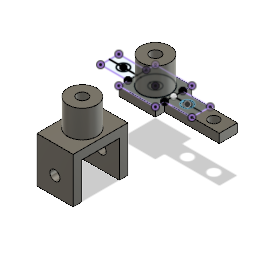
AluminumFesting v3 (Autodesk Fusion 360 design; units mm, degrees)
Autodesk Fusion 360 part; units mm, degrees
sketch "Sketch1" plane through (0, 0, 0) normal (0, 1, 0) x (1, 0, 0)
  line L0 (-10, 10) -> (10, 10)
  line L1 (10, 10) -> (10, -10)
  line L2 (10, -10) -> (-10, -10)
  line L3 (-10, -10) -> (-10, 10)
  line L4 (-10, 10) -> (10, -10) construction
  line L5 (10, 10) -> (-10, -10) construction
  line L6 (-10, -5) -> (-25, -5)
  line L7 (-25, -5) -> (-25, 5)
  line L8 (-25, 5) -> (-10, 5)
  line L9 (-10, 5) -> (-10, -5)
  line L10 (10, -5) -> (25, -5)
  line L11 (25, -5) -> (25, 5)
  line L12 (25, 5) -> (10, 5)
  line L13 (10, 5) -> (10, -5)
  dimension "d1" = 20
  constraint horizontal L0
  constraint perpendicular L0 L1
  constraint parallel L0 L2
  constraint parallel L1 L3
  constraint coincident L4 origin
  constraint coincident L5 origin
  constraint horizontal L6
  constraint vertical L7
  constraint horizontal L8
  constraint vertical L9
  constraint coincident L3 L6.start
  constraint horizontal L10
  constraint vertical L11
  constraint horizontal L12
  constraint vertical L13
  constraint coincident L1 L10.start
  measures "d1" distance of L0.end L1.end
extrude "Extrude1" add sketch "Sketch1" along normal blind 5 makes body 1
sketch "Sketch2" plane through (0, 5, 0) normal (0, 1, 0) x (-1, 0, 0)
  line L0 (-10, 5) -> (-25, 5)
  line L1 (-25, 5) -> (-25, -5)
  line L2 (-25, -5) -> (-10, -5)
  line L3 (-10, -5) -> (-10, -10)
  line L4 (-10, -10) -> (10, -10)
  line L5 (10, -10) -> (10, -5)
  line L6 (10, -5) -> (25, -5)
  line L7 (25, -5) -> (25, 5)
  line L8 (25, 5) -> (10, 5)
  line L9 (10, 5) -> (10, 10)
  line L10 (10, 10) -> (-10, 10)
  line L11 (-10, 10) -> (-10, 5)
  line L12 (10, -5) -> (10, 5)
  line L13 (-10, 5) -> (-10, -5)
  line L14 (10, 0) -> (25, 0)
  line L15 (-10, 0) -> (-25, 0)
  circle A0 centre (17.5, 0) radius 2.75
  circle A1 centre (-17.5, 0) radius 2.75
  circle A2 centre (0, 0) radius 2.9
  circle A3 centre (0, 0) radius 8
  dimension "d4" = 5.5
  dimension "d5" = 5.5
  dimension "d6" = 5.8
  dimension "d7" = 16
  constraint coincident L5.end L6.start
  constraint coincident L8.end L9.start
  constraint coincident L0.start L11.end
  constraint coincident L2.end L3.start
  constraint midpoint L12 L14.start
  constraint midpoint L7 L14.end
  constraint midpoint L1 L15.end
  constraint perpendicular L1 L15
  constraint midpoint L14 A0.centre
  constraint midpoint L15 A1.centre
  constraint coincident A2.centre A3.centre
  measures "d4" diameter of A0
  measures "d5" diameter of A1
  measures "d6" diameter of A2
  measures "d7" diameter of A3
extrude "Extrude2" cut sketch "Sketch2" against normal blind 12 contours L15 A1 | L15 A1 | L14 A0 | L14 A0 bodies 1
extrude "Extrude3" add sketch "Sketch2" along normal blind 15 contours A3 bodies 1
copy_body "CopyPasteBodies1" bodies 1 makes body 2
move_body "Move1" bodies 2 to x (1, 0, 0) y (0, 1, 0) z (0, 0, 1) at (0, 0, 40)
sketch "Sketch3" plane through (0, 5, 0) normal (0, 1, 0) x (-1, 0, 0)
  line L0 (-10, 45) -> (-25, 45)
  line L1 (-25, 45) -> (-25, 35)
  line L2 (-25, 35) -> (-10, 35)
  line L3 (-10, 35) -> (-10, 30)
  line L4 (-10, 30) -> (10, 30)
  line L5 (10, 30) -> (10, 35)
  line L6 (10, 35) -> (25, 35)
  line L7 (25, 35) -> (25, 45)
  line L8 (25, 45) -> (10, 45)
  line L9 (10, 45) -> (10, 50)
  line L10 (10, 50) -> (-10, 50)
  line L11 (-10, 50) -> (-10, 45)
  circle A0 centre (-17.5, 40) radius 2.75
  circle A1 centre (17.5, 40) radius 2.75
  circle A2 centre (0, 40) radius 8
  line L12 (-10, 45) -> (-10, 35)
  line L13 (10, 45) -> (10, 35)
  constraint coincident L0.start L11.end
  constraint coincident L2.end L3.start
  constraint coincident L8.end L9.start
  constraint coincident L5.end L6.start
extrude "Extrude4" cut sketch "Sketch3" against normal blind 25 contours L0 L1 L2 L12 | L6 L7 L8 L13 bodies 2
sketch "Sketch4" plane through (0, 0, 50) normal (0, 0, 1) x (1, 0, 0)
  line L0 (-10, 0) -> (10, 0)
  line L1 (10, 0) -> (10, 5)
  line L2 (10, 5) -> (-10, 5)
  line L3 (-10, 5) -> (-10, 0)
  line L4 (-10, 5) -> (10, 5)
  line L5 (10, 5) -> (10, -20)
  line L6 (10, -20) -> (-10, -20)
  line L7 (-10, -20) -> (-10, 5)
  dimension "d14" = 25
  constraint horizontal L4
  constraint vertical L5
  constraint horizontal L6
  constraint vertical L7
  constraint coincident L2.end L3.start
  measures "d14" distance of L2.end L6.end
extrude "Extrude5" add sketch "Sketch4" along normal blind 5 bodies 2
sketch "Sketch5" plane through (0, 0, 30) normal (0, 0, -1) x (-1, 0, 0)
  line L0 (-10, 0) -> (10, 0)
  line L1 (10, 0) -> (10, 5)
  line L2 (10, 5) -> (-10, 5)
  line L3 (-10, 5) -> (-10, 0)
  line L4 (-10, 5) -> (10, 5)
  line L5 (10, 5) -> (10, -20)
  line L6 (10, -20) -> (-10, -20)
  line L7 (-10, -20) -> (-10, 5)
  constraint horizontal L4
  constraint vertical L5
  constraint horizontal L6
  constraint vertical L7
  constraint coincident L2.end L3.start
extrude "Extrude6" add sketch "Sketch5" along normal blind 5 bodies 2
sketch "Sketch6" plane through (0, 0, 25) normal (0, 0, -1) x (-1, 0, 0)
  line L0 (-10, -20) -> (10, -20)
  line L1 (10, -20) -> (10, 5)
  line L2 (10, 5) -> (-10, 5)
  line L3 (-10, 5) -> (-10, -20)
  line L4 (0, -20) -> (0, -10)
  circle A0 centre (0, -10) radius 2.75
  dimension "d19" = 10
  dimension "d20" = 5.5
  constraint midpoint L0 L4.start
  constraint perpendicular L0 L4
  constraint coincident L4.end A0.centre
  measures "d19" distance of L4.start L4.end
  measures "d20" diameter of A0
sketch "Sketch7" plane through (0, 0, 55) normal (0, 0, 1) x (1, 0, 0)
  line L0 (-10, -20) -> (10, -20)
  line L1 (10, -20) -> (10, 5)
  line L2 (10, 5) -> (-10, 5)
  line L3 (-10, 5) -> (-10, -20)
  line L4 (0, -20) -> (0, -10)
  circle A0 centre (0, -10) radius 2.75
  dimension "d21" = 5.5
  constraint midpoint L0 L4.start
  constraint perpendicular L0 L4
  constraint coincident L4.end A0.centre
  measures "d21" diameter of A0
extrude "Extrude7" cut sketch "Sketch7" against normal blind 10 contours A0 bodies 2
extrude "Extrude8" cut sketch "Sketch6" against normal blind 10 contours A0 bodies 2
sketch "Sketch8" plane through (0, 5, 0) normal (0, 1, 0) x (-1, 0, 0)
  circle A0 centre (0, 40) radius 2.9
  circle A1 centre (0, 40) radius 2.9
  dimension "d26" = 5.8
  constraint concentric A0 A1
  measures "d26" diameter of A1
extrude "Extrude9" add sketch "Sketch8" along normal blind 15 bodies 2
extrude "Extrude10" cut 1 faces at (0.0685, -17.5808, 50) along direction (0, 0, 1) blind 0.3 on bodies 2 bodies 2
extrude "Extrude11" cut 1 faces at (-0.0685, -17.5808, 30) along direction (0, 0, -1) blind 0.3 on bodies 2 bodies 2
extrude "Extrude12" add sketch "Sketch2" against normal blind 5 separate body contours L0 L1 L13 L15 A1 | L3 L4 L5 L9 L10 L11 L12 L13 | L1 L2 L13 L15 A1 | A2 | A3 makes body 3
sketch "Sketch9" plane through (0, 20, 0) normal (0, 1, 0) x (-1, 0, 0)
  circle A0 centre (0, 40) radius 8
  circle A1 centre (0, 40) radius 2.9
  dimension "d35" = 5.8
  constraint concentric A0 A1
  measures "d35" diameter of A1
extrude "Extrude13" cut sketch "Sketch9" against normal blind 15 contours A1 bodies 2
extrude "Extrude14" add sketch "Sketch2" along normal blind 15 contours A3 bodies 3
move_face "OffsetFaces1" offset 15 1 faces at (25, 3.3333, 1.6667) on bodies 3
sketch "Sketch10" plane through (0, 5, 0) normal (0, 1, 0) x (-1, 0, 0)
  line L0 (10, -10) -> (10, 10)
  line L1 (10, 10) -> (-10, 10)
  line L2 (-10, 10) -> (-10, 5)
  line L3 (-10, 5) -> (-40, 5)
  line L4 (-40, 5) -> (-40, -5)
  line L5 (-40, -5) -> (-10, -5)
  line L6 (-10, -5) -> (-10, -10)
  line L7 (-10, -10) -> (10, -10)
  circle A0 centre (-17.5, 0) radius 2.75
  circle A1 centre (0, 0) radius 8
  line L8 (-40, 0) -> (-32, 0)
  circle A2 centre (-32, 0) radius 2.8
  dimension "d41" = 8
  dimension "d42" = 5.6
  constraint midpoint L4 L8.start
  constraint perpendicular L4 L8
  constraint coincident L8.end A2.centre
  measures "d41" distance of L8.start L8.end
  measures "d42" diameter of A2
extrude "Extrude15" cut sketch "Sketch10" against normal blind 10 contours A2 bodies 3
hidden bodies 1
